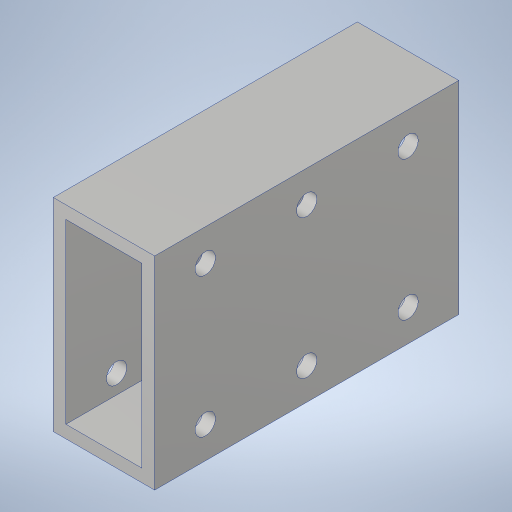
# Autodesk Inventor part: EL2-S-003
Saved by Autodesk Inventor 2023.4 (Build 274418000, 418)
## iProperties
RuleStatus: InUse
Created: 2025-01-13
Part Number: EL2-S-003
Material: Aluminum 6061
Document SubType Name: Modeling
Designer: mavericks
Mass: 304.185 g
Surface Area: 718.547 cm^2
Volume: 112.661 cm^3
Density: 2.7 g/cm^3
Appearance: Aluminum - Flat
AfterDocNew0: SHOW
AfterDocOpen0: SHOW
Author: mavericks
Autodesk Inventor part; units mm, degrees
ref_plane "YZ Plane" through (0, 0, 0) normal (1, 0, 0) x (0, 1, 0)
ref_plane "XZ Plane" through (0, 0, 0) normal (0, 1, 0) x (-1, 0, 0)
ref_plane "XY Plane" through (0, 0, 0) normal (0, 0, 1) x (1, 0, 0)
sketch "Sketch1" plane through (0, 0, 0) normal (0, 0, 1) x (1, 0, 0)
  line L0 (-12.7, -25.4) -> (12.7, -25.4)
  line L1 (12.7, -25.4) -> (12.7, 25.4)
  line L2 (12.7, 25.4) -> (-12.7, 25.4)
  line L3 (-12.7, 25.4) -> (-12.7, -25.4)
  line L4 (-12.7, -25.4) -> (12.7, 25.4) construction
  line L5 (12.7, -25.4) -> (-12.7, 25.4) construction
  line L6 (-9.525, 22.225) -> (9.525, 22.225)
  line L7 (9.525, 22.225) -> (9.525, -22.225)
  line L8 (9.525, -22.225) -> (-9.525, -22.225)
  line L9 (-9.525, -22.225) -> (-9.525, 22.225)
  point P0 (0, 0)
  dimension "width" = 25.4
  dimension "height" = 50.8
  dimension "thickness" = 3.175
  constraints: 20 end point, 4 parallel, 2 midpoint, 2 perpendicular, 1 horizontal, 3 other
  measures "width" distance of L2.end L1.end
  measures "height" distance of L1.end L0.end
  measures "thickness" distance between parallel lines of L2 L6
extrude "Extrusion1" add sketch "Sketch1" along normal mid plane 76.2
sketch "Sketch2" plane through (12.7, -25.4, 38.1) normal (1, 0, 0) x (0, 0, -1)
  line L0 (76.2, 50.8) -> (0, 50.8) construction
  line L1 (0, 0) -> (0, 50.8) construction
  line L2 (76.2, 0) -> (0, 0) construction
  line L3 (76.2, 50.8) -> (76.2, 0) construction
  circle A0 centre (63.5, 42.8625) radius 4.7625 construction
  line L4 (0, 47.625) -> (76.2, 47.625) construction
  circle A1 centre (63.5, 7.9375) radius 4.7625 construction
  line L5 (0, 3.175) -> (76.2, 3.175) construction
  point P0 (38.1, 25.4)
  point P1 (38.1, 42.8625)
  point P2 (38.1, 7.9375)
  point P3 (12.7, 42.8625)
  point P4 (12.7, 7.9375)
  point P5 (-12.7, 42.8625)
  point P6 (-12.7, 7.9375)
  point P7 (-38.1, 42.8625)
  point P8 (-38.1, 7.9375)
  point P9 (-63.5, 42.8625)
  point P10 (-63.5, 7.9375)
  point P11 (-88.9, 42.8625)
  point P12 (-88.9, 7.9375)
  point P13 (-114.3, 42.8625)
  point P14 (-114.3, 7.9375)
  point P15 (-139.7, 42.8625)
  point P16 (-139.7, 7.9375)
  point P17 (-165.1, 42.8625)
  point P18 (-165.1, 7.9375)
  dimension "d5" = 9.525
  dimension "d6" = 9.525
  dimension "d7" = 12.7
  dimension "d10" = 25.4
  constraints: 4 coincident, 2 centre point, 2 tangent, 1 horizontal, 1 vertical alignment, 18 other
  measures "d5" diameter of A0
  measures "d6" diameter of A1
  measures "d7" distance from line of L3 A0.centre
  measures "d10" distance of point (63.5, 42.863) point (38.1, 42.863)
hole "Hole1" at (12.7, 17.4625, -25.4) at (12.7, -17.4625, -25.4) at (12.7, 17.4625, 0) at (12.7, -17.4625, 0) at (12.7, 17.4625, 25.4) at (12.7, -17.4625, 25.4) at (12.7, 17.4625, 50.8) at (12.7, -17.4625, 50.8) at (12.7, 17.4625, 76.2) at (12.7, -17.4625, 76.2) at (12.7, 17.4625, 101.6) at (12.7, -17.4625, 101.6) at (12.7, 17.4625, 127) at (12.7, -17.4625, 127) at (12.7, 17.4625, 152.4) at (12.7, -17.4625, 152.4) at (12.7, 17.4625, 177.8) at (12.7, -17.4625, 177.8) at (12.7, 17.4625, 203.2) at (12.7, -17.4625, 203.2) direction (-1, 0, 0) diameter 5.1054 end through all clearance for "Flat Head Machine Screw (82)" size "#10" standard "Ansi Unified Screw Threads"
body "Solid1"
